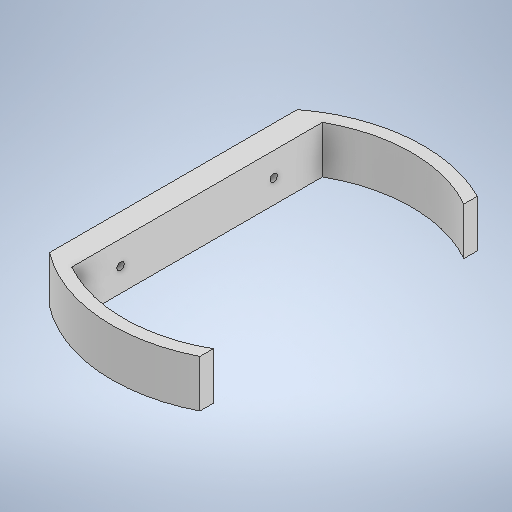
# Autodesk Inventor part: Roof_Mount
Saved by Autodesk Inventor 2025 (Build 290162010, 162A)
## iProperties
Created: 2024-07-25
Part Number: Roof_Mount
Material: Generic
Document SubType Name: Modeling
Designer: vncnt
Density: 1 g/cm^3
Appearance: Default
Author: vncnt
Autodesk Inventor part; units mm, degrees
ref_plane "YZ Plane" through (0, 0, 0) normal (1, 0, 0) x (0, 1, 0)
ref_plane "XZ Plane" through (0, 0, 0) normal (0, 1, 0) x (-1, 0, 0)
ref_plane "XY Plane" through (0, 0, 0) normal (0, 0, 1) x (1, 0, 0)
sketch "Sketch5" plane through (0, 0, 0) normal (0, 1, 0) x (-1, 0, 0)
  line L0 (-19, -37.2559) -> (-19, 37.2559)
  line L1 (19, -33.653) -> (19, 33.653)
  line L2 (25.35, -33.2623) -> (25.35, 33.2623)
  arc A0 (-19, -37.2559) -> (25.35, -33.2623) centre (0, 0) ccw
  arc A1 (25.35, 33.2623) -> (-19, 37.2559) centre (0, 0) ccw
  arc A2 (-19, -33.653) -> (19, -33.653) centre (0, 0) ccw
  arc A3 (19, 33.653) -> (-19, 33.653) centre (0, 0) ccw
  dimension "d50" = 19
  dimension "d51" = 19
  dimension "d52" = 6.35
  dimension "d53" = 38.6461
  dimension "d54" = 41.8211
  constraints: 8 point on circle, 6 end point, 4 centre point, 2 coincident, 2 point on line, 2 vertical, 1 parallel
  measures "d50" distance from line of L0 point (0, 0)
  measures "d51" distance from line of point (0, 0) L1
  measures "d52" distance between parallel lines of L1 L2
  measures "d53" radius of A3
  measures "d54" radius of A1
extrude "Extrusion4" add sketch "Sketch5" along normal blind 12.7 contours L0 A2 L1 A3 A1 L2 A0
sketch "Sketch6" plane through (-25.35, 0, -33.2623) normal (-1, 0, 0) x (0, 0, 1)
  line L0 (0, 0) -> (0, 12.7) projected
  line L1 (0, 12.7) -> (66.5246, 12.7) projected
  line L2 (66.5246, 0) -> (66.5246, 12.7) projected
  point P0 (33.2623, 0)
  point P1 (12.7, 6.35)
  point P2 (53.8246, 6.35)
  dimension "d57" = 12.7
  dimension "d58" = 6.35
  dimension "d59" = 6.35
  dimension "d60" = 12.7
  measures "d57" distance from line of L0 point (12.7, 6.35)
  measures "d58" distance from line of L1 point (12.7, 6.35)
  measures "d59" distance from line of L1 point (53.825, 6.35)
  measures "d60" distance from line of L2 point (53.825, 6.35)
hole "Hole2" at (-25.35, 6.35, -20.5623) at (-25.35, 6.35, 20.5623) direction (1, 0, 0) diameter 2 end through all
body "Solid2"
